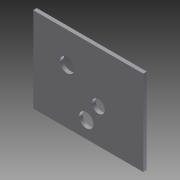
# Autodesk Inventor part: tiltBoxBase
Saved by Autodesk Inventor 2012 (Build 160160000, 160)
## iProperties
Created: 2014-06-12
Part Number: tiltBoxBase
Material: Default
Document SubType Name: Modeling
Designer: Byron
Density: 1 g/cm^3
Author: Byron
Autodesk Inventor part; units mm, degrees
ref_plane "YZ Plane" through (0, 0, 0) normal (1, 0, 0) x (0, 1, 0)
ref_plane "XZ Plane" through (0, 0, 0) normal (0, 1, 0) x (-1, 0, 0)
ref_plane "XY Plane" through (0, 0, 0) normal (0, 0, 1) x (1, 0, 0)
sketch "Sketch1" plane through (0, 0, 0) normal (0, 0, 1) x (1, 0, 0)
  circle A0 centre (-24.464, 35.97) radius 1.27 projected
  circle A1 centre (31.416, 0) radius 3.175 projected
  line L0 (-56.214, -50.8) -> (-56.214, 50.8) projected
  line L1 (97.7735, -50.8) -> (-56.214, -50.8) projected
  line L2 (97.7735, 50.8) -> (97.7735, -50.8) projected
  line L3 (-56.214, 50.8) -> (97.7735, 50.8) projected
  circle A2 centre (9.7431, -32.1205) radius 12.7 projected
  circle A3 centre (-24.464, 35.97) radius 12.7 projected
  circle A4 centre (31.416, 0) radius 11.4366
  line L4 (111.6872, -61.5577) -> (-85.1628, -61.5577)
  line L5 (-85.1628, -61.5577) -> (-85.1628, 90.8423)
  line L6 (-85.1628, 90.8423) -> (111.6872, 90.8423)
  line L7 (111.6872, 90.8423) -> (111.6872, -61.5577)
  point P0 (0, 0)
  dimension "d0" = 196.85
  dimension "d1" = 152.4
  constraints: 8 end point, 2 parallel, 1 centre point, 1 horizontal, 1 perpendicular
  measures "d0" distance of L4.start L4.end
  measures "d1" distance of L6.end L4.start
extrude "Extrusion1" add sketch "Sketch1" along normal blind 6.35 contours L0 L3 L2 L1 | L4 L5 L6 L7
body "Solid1"
